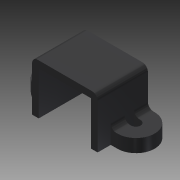
# Autodesk Inventor part: Mount_Motor
Saved by Autodesk Inventor 2013 (Build 170138000, 138)
## iProperties
Created: 2015-07-06
Part Number: Mount_Motor
Material: Nylon 6/6
Document SubType Name: Modeling
Designer: Kyle
Density: 1.13 g/cm^3
Mass: 0.929978 g
Surface Area: 11.726 cm^2
Volume: 0.82299 cm^3
Author: Kyle
Autodesk Inventor part; units mm, degrees
ref_plane "YZ Plane" through (0, 0, 0) normal (1, 0, 0) x (0, 1, 0)
ref_plane "XZ Plane" through (0, 0, 0) normal (0, 1, 0) x (-1, 0, 0)
ref_plane "XY Plane" through (0, 0, 0) normal (0, 0, 1) x (1, 0, 0)
sketch "Sketch1" plane through (0, 0, 0) normal (0, 0, 1) x (1, 0, 0)
  line L0 (0, 2.9972) -> (0, 11.5062)
  line L1 (0, 11.5062) -> (15.0114, 11.5062)
  line L2 (15.0114, 11.5062) -> (15.0114, 2.9972)
  line L3 (13.5001, 0) -> (13.5001, 9.9949)
  line L4 (13.5001, 9.9949) -> (1.5113, 9.9949)
  line L5 (1.5113, 9.9949) -> (1.5113, 0)
  line L6 (15.0114, 2.9972) -> (20.8026, 2.9972)
  line L7 (20.8026, 2.9972) -> (20.8026, 0)
  line L8 (20.8026, 0) -> (15.0113, 0)
  line L9 (15.0113, 0) -> (13.5001, 0)
  line L10 (0, 0) -> (-5.7912, 0)
  line L11 (-5.7912, 2.9972) -> (0, 2.9972)
  line L12 (0, 0) -> (1.5113, 0)
  line L13 (-5.7912, 2.9972) -> (-5.7912, 0)
  dimension "d0" = 11.5062
  dimension "d2" = 15.0114
  dimension "d3" = 11.9888
  dimension "d4" = 0
  dimension "d5" = 0
  dimension "d6" = 0
  dimension "d7" = 5.7912
  dimension "d8" = 5.7912
  dimension "d9" = 2.9972
  dimension "d10" = 2.9972
  constraints: 28 end point, 6 perpendicular, 3 parallel, 2 vertical, 1 coincident, 1 collinear, 1 horizontal
  measures "d0" distance of L10.start L0.end
  measures "d2" distance of L0.end L1.end
  measures "d3" distance of L3.end L4.end
  measures "d4" vertical distance of point (0, 0) L5.end
  measures "d5" vertical distance of point (0, 0) L3.start
  measures "d6" vertical distance of point (0, 0) L8.end
  measures "d7" distance of L2.end L6.end
  measures "d8" distance of L11.start L0.start
  measures "d9" distance of L6.end L7.end
  measures "d10" distance from line of point (0, 0) L11
extrude "Extrusion1" add sketch "Sketch1" along normal blind 11.5062
sketch "Sketch2" plane through (0, 0, 11.5062) normal (0, 0, 1) x (1, 0, 0)
  line L0 (15.0114, 2.9972) -> (20.8026, 2.9972)
  line L1 (20.8026, 2.9972) -> (20.8026, 0)
  line L2 (20.8026, 0) -> (15.0114, 0)
  line L3 (15.0114, 0) -> (15.0114, 2.9972)
  line L4 (0, 2.9972) -> (-5.7912, 2.9972)
  line L5 (-5.7912, 2.9972) -> (-5.7912, 0)
  line L6 (-5.7912, 0) -> (0, 0)
  line L7 (0, 0) -> (0, 2.9972)
  point P0 (0, 0)
  constraints: 16 end point, 4 parallel, 2 horizontal, 2 perpendicular
extrude "Extrusion2" cut sketch "Sketch2" against normal blind 2.9972
sketch "Sketch3" plane through (15.0114, 2.9972, 0) normal (0, 1, 0) x (1, 0, 0)
  line L0 (0, 0) -> (0, -8.509) projected
  arc A0 (1.4999, -5.3467) -> (1.4325, -3.1643) centre (1.4986, -4.2545) ccw
  arc A1 (-16.51, -3.1604) -> (-16.51, -5.3486) centre (-16.51, -4.2545) ccw
  line L1 (-15.0114, 0) -> (-15.0114, -11.5062) projected
  line L2 (-16.51, -3.1604) -> (-15.0114, -3.1604)
  line L3 (-15.0114, -3.1604) -> (-15.0114, -5.3486)
  line L4 (-15.0114, -5.3486) -> (-16.51, -5.3486)
  line L5 (1.4325, -3.1643) -> (0, -3.1643)
  line L6 (0, -3.1643) -> (0, -5.3486)
  line L7 (0, -5.3486) -> (1.4999, -5.3467)
  dimension "d15" = 2.1844
  dimension "d17" = 1.4986
  dimension "d18" = 1.4986
  constraints: 12 end point, 4 point on circle, 4 point on line, 3 tangent, 2 centre point, 1 parallel, 1 perpendicular
  measures "d15" diameter of A0
  measures "d17" distance from line of A0.centre L0
  measures "d18" distance from line of L1 A1.centre
extrude "Extrusion3" cut sketch "Sketch3" against normal blind 50.8
fillet "Fillet1" radius 4.2545 4 edges at (20.8026, 1.4986, 8.509) (20.8026, 1.4986, 0) (-5.7912, 1.4986, 8.509) (-5.7912, 1.4986, 0)
fillet "Fillet2" radius 1.27 6 edges at (0, 2.9972, 1.5802) (0, 2.9972, 6.9288) (0, 11.5062, 5.7531) (15.0114, 11.5062, 5.7531) (15.0114, 2.9972, 1.5822) (15.0114, 2.9972, 6.9288)
body "Solid1"
